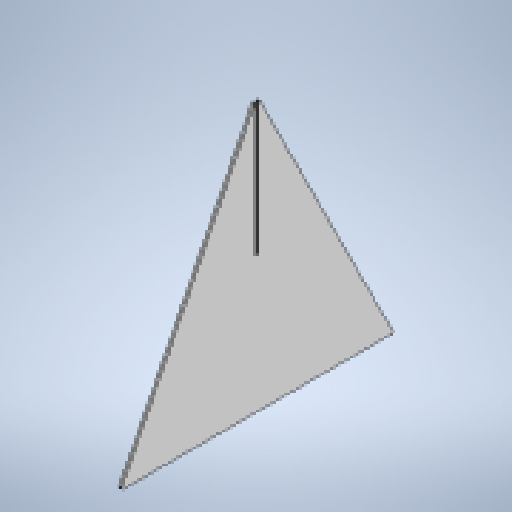
# Autodesk Inventor part: MSC 205 CONE BLADE
Saved by Autodesk Inventor 2025.1 (Build 291241020, 241B)
## iProperties
Created: 2025-01-15
Part Number: MSC 205 CONE BLADE
Material: Stainless Steel
Document SubType Name: Sheet Metal
Designer: pokla
Density: 8 g/cm^3
Sheet Metal Rule: AISI304 3mm Die 32
Appearance: Default
Author: pokla
Autodesk Inventor part; units mm, degrees
ref_plane "YZ Plane" through (0, 0, 0) normal (1, 0, 0) x (0, 1, 0)
ref_plane "XZ Plane" through (0, 0, 0) normal (0, 1, 0) x (-1, 0, 0)
ref_plane "XY Plane" through (0, 0, 0) normal (0, 0, 1) x (1, 0, 0)
sketch "Sketch1" plane through (0, 0, 0) normal (1, 0, 0) x (0, 1, 0)
  line L0 (150, 0) -> (-150, 0)
  line L1 (0, 0) -> (0, 300)
  line L2 (0, 300) -> (150, 0)
  line L3 (0, 300) -> (-150, 0)
  dimension "d0" = 300
  dimension "d1" = 300
  measures "d0" distance of L0.start L0.end
  measures "d1" distance of L1.start L1.end
extrude "Plate1" add sketch "Sketch1" along normal mid plane 3
sketch "Sketch2" plane through (-1.5, 0, 0) normal (-1, 0, 0) x (0, 0, 1)
  line L0 (300, -1.6) -> (149, -1.6)
  line L1 (149, -1.6) -> (149, 1.6)
  line L2 (149, 1.6) -> (300, 1.6)
  line L3 (300, 1.6) -> (300, -1.6)
  point P0 (0, 0)
  point P1 (300, 0)
  point P2 (300, 0)
  dimension "d3" = 3.2
  dimension "d4" = 151
  constraints: 8 end point, 2 parallel, 1 coincident, 1 horizontal, 1 midpoint, 1 perpendicular
  measures "d3" distance of L2.end L0.start
  measures "d4" distance of L0.start L0.end
extrude "Extrusion1" cut sketch "Sketch2" against normal through all
chamfer "Corner Chamfer1" distance 2 angle 45 4 edges at (0, -1.6, 296.8) (0, 1.6, 296.8) (0, 150, 0) (0, -150, 0)
equation "\"d2\" = Thickness"
equation "\"BendReliefWidth\" = Thickness"
equation "\"BendReliefDepth\" = 0.5 * Thickness"
equation "\"CornerReliefSize\" = 4 * Thickness"
equation "\"MinimumRemnant\" = 2 * Thickness"
equation "\"TransitionRadius\" = BendRadius"
equation "\"JacobiRadiusSize\" = BendRadius"
equation "\"GapSize\" = Thickness"
equation "\"Thickness\" = 3"
equation "\"BendRadius\" = 5"
body "Solid1"
